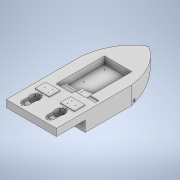
# Autodesk Inventor part: MainBody
Saved by Autodesk Inventor 2020.1 (Build 241239000, 239)
## iProperties
Created: 2021-12-15
Part Number: MainBody
Material: Generic
Document SubType Name: Modeling
Designer: OEM
Density: 1 g/cm^3
Appearance: Default
Author: OEM
Autodesk Inventor part; units mm, degrees
ref_plane "YZ Plane" through (0, 0, 0) normal (1, 0, 0) x (0, 1, 0)
ref_plane "XZ Plane" through (0, 0, 0) normal (0, 1, 0) x (-1, 0, 0)
ref_plane "XY Plane" through (0, 0, 0) normal (0, 0, 1) x (1, 0, 0)
sketch "Sketch1" plane through (0, 0, 0) normal (0, 1, 0) x (-1, 0, 0)
  line L0 (28.25, 20.4) -> (-28.25, 20.4) construction
  line L1 (-28.25, 20.4) -> (-28.25, -65.2) construction
  line L2 (-28.25, -65.2) -> (28.25, -65.2) construction
  line L3 (28.25, -65.2) -> (28.25, 20.4) construction
  line L4 (28.25, 20.4) -> (-28.25, -65.2) construction
  line L5 (-28.25, 20.4) -> (28.25, -65.2) construction
  line L6 (0, 600.8) -> (0, -638.2) construction
  spline S0 degree 2 poles (70, -42.8) (58.3679, -124.7541) (0, -160.2) knots 0 0 0 1 1 1
  line L7 (70, -42.8) -> (70, 157.2)
  spline S1 degree 2 poles (-70, -42.8) (-58.3679, -124.7541) (0, -160.2) knots 0 0 0 1 1 1
  line L8 (-70, -42.8) -> (-70, 157.2)
  line L9 (70, 87.2) -> (-70, 87.2)
  line L10 (0, 87.2) -> (70, 157.2) construction
  line L11 (0, 157.2) -> (70, 87.2) construction
  circle A0 centre (35, 122.2) radius 12.5
  line L12 (0, 87.2) -> (-70, 157.2) construction
  line L13 (0, 157.2) -> (-70, 87.2) construction
  circle A1 centre (-35, 122.2) radius 12.5
  line L14 (-38.25, 30.4) -> (38.25, 30.4)
  line L15 (38.25, 30.4) -> (38.25, -75.2)
  line L16 (38.25, -75.2) -> (-38.25, -75.2)
  line L17 (-38.25, -75.2) -> (-38.25, 30.4)
  line L18 (-38.25, 30.4) -> (38.25, -75.2) construction
  line L19 (38.25, 30.4) -> (-38.25, -75.2) construction
  line L20 (-6.75, 50.4) -> (38.25, 50.4)
  line L21 (38.25, 50.4) -> (38.25, 30.4)
  line L22 (-6.75, 30.4) -> (-6.75, 50.4)
  circle A2 centre (24.5, -61.7) radius 1.125
  circle A3 centre (-24.5, -61.7) radius 1.125
  line L23 (-24.5, -61.7) -> (24.5, -61.7) construction
  line L24 (-24.5, -32.7) -> (24.5, -32.7) construction
  line L25 (-24.5, -32.7) -> (-24.5, -61.7) construction
  line L26 (24.5, -32.7) -> (24.5, -61.7) construction
  circle A4 centre (24.5, -3.7) radius 1.125
  circle A5 centre (-24.5, -3.7) radius 1.125
  line L27 (-24.5, -3.7) -> (24.5, -3.7) construction
  line L28 (-24.5, -32.7) -> (-24.5, -3.7) construction
  line L29 (24.5, -32.7) -> (24.5, -3.7) construction
  line L30 (-6.75, 30.4) -> (-38.25, 30.4)
  line L31 (-38.25, 30.4) -> (-38.25, 50.4) construction
  line L32 (-38.25, 50.4) -> (-6.75, 50.4) construction
  line L33 (-6.75, 50.4) -> (-6.75, 30.4)
  line L34 (-6.75, 30.4) -> (-37.23, 30.4)
  line L35 (-37.23, 30.4) -> (-37.23, 51.99)
  line L36 (-37.23, 51.99) -> (-6.75, 51.99)
  line L37 (-6.75, 51.99) -> (-6.75, 30.4)
  circle A6 centre (-34.69, 32.94) radius 0.75
  circle A7 centre (-20.085, 49.45) radius 0.75
  line L38 (-45, 112.2) -> (-45, 152)
  line L39 (-45, 152) -> (-25, 152)
  line L40 (-25, 112.2) -> (-25, 108.45) construction
  line L41 (-25, 108.45) -> (-45, 108.45) construction
  line L42 (-45, 108.45) -> (-45, 112.2) construction
  line L43 (-25, 112.2) -> (-25, 152)
  line L44 (-45, 112.2) -> (-25, 112.2)
  line L45 (-25, 152) -> (-45, 152)
  line L46 (-45, 152) -> (-45, 155.75) construction
  line L47 (-45, 155.75) -> (-25, 155.75) construction
  line L48 (-25, 155.75) -> (-25, 152) construction
  line L49 (70, 157.2) -> (-70, 157.2) construction
  line L50 (-70, 157.2) -> (-70, 167.2)
  line L51 (-70, 167.2) -> (70, 167.2)
  line L52 (70, 167.2) -> (70, 157.2)
  line L53 (-35, 108.45) -> (-35, 155.75) construction
  circle A8 centre (-30, 155.75) radius 2
  line L54 (-25, 132.1) -> (-45, 132.1) construction
  circle A9 centre (-40, 155.75) radius 2
  circle A10 centre (-30, 108.45) radius 2
  circle A11 centre (-40, 108.45) radius 2
  line L55 (45, 112.2) -> (45, 152)
  line L56 (45, 152) -> (25, 152)
  line L57 (25, 112.2) -> (25, 152)
  line L58 (45, 112.2) -> (25, 112.2)
  line L59 (45, 152) -> (45, 155.75) construction
  line L60 (45, 155.75) -> (25, 155.75) construction
  line L61 (25, 155.75) -> (25, 152) construction
  line L62 (35, 108.45) -> (35, 155.75) construction
  circle A12 centre (30, 155.75) radius 2
  circle A13 centre (40, 155.75) radius 2
  circle A14 centre (30, 108.45) radius 2
  circle A15 centre (40, 108.45) radius 2
  line L63 (45, 108.45) -> (25, 108.45) construction
  line L64 (45, 108.45) -> (45, 112.2) construction
  line L65 (25, 108.45) -> (25, 112.2) construction
  line L66 (-72.4135, -25.7958) -> (-67.5865, -59.8042) construction
  arc A16 (-71.5687, -29.1646) -> (-67.7125, -56.3334) centre (186.925, -6.3334) ccw construction
  line L67 (-15, 102.2) -> (-55, 102.2)
  line L68 (-55, 102.2) -> (-55, 72.2)
  line L69 (-55, 72.2) -> (-15, 72.2)
  line L70 (-15, 72.2) -> (-15, 102.2)
  line L71 (-15, 102.2) -> (-55, 72.2) construction
  line L72 (-55, 102.2) -> (-15, 72.2) construction
  line L73 (15, 102.2) -> (55, 102.2)
  line L74 (55, 102.2) -> (55, 72.2)
  line L75 (55, 72.2) -> (15, 72.2)
  line L76 (15, 72.2) -> (15, 102.2)
  circle A17 centre (26.8629, 81.1136) radius 0.75
  circle A18 centre (42.4108, 87.2) radius 0.75
  circle A19 centre (26.8629, 93.2864) radius 0.75
  circle A20 centre (-26.8629, 81.1136) radius 0.75
  circle A21 centre (-42.4108, 87.2) radius 0.75
  circle A22 centre (-26.8629, 93.2864) radius 0.75
  line L77 (-26.75, 30.4) -> (-26.75, 33.4)
  line L78 (-26.75, 33.4) -> (-37.23, 33.4) construction
  line L79 (-14.75, 33.4) -> (-14.75, 51.99)
  line L80 (-14.75, 33.4) -> (-26.75, 33.4)
  line L81 (-14.75, 33.4) -> (-14.75, 30.4) construction
  line L82 (-14.75, 33.4) -> (-6.75, 33.4) construction
  line L83 (-37.23, 50.99) -> (-62.23, 50.99)
  line L84 (-37.23, 40.99) -> (-62.23, 40.99)
  line L85 (-62.23, 50.99) -> (-62.23, 40.99)
  line L86 (-35.6, 152) -> (-35.6, 160)
  line L87 (-35.6, 160) -> (-35, 160)
  line L88 (-34.4, 152) -> (-34.4, 160)
  line L89 (-34.4, 160) -> (-35, 160)
  line L90 (-35.6, 112.2) -> (-35.6, 104.2)
  line L91 (-35.6, 104.2) -> (-35, 104.2)
  line L92 (-34.4, 112.2) -> (-34.4, 104.2)
  line L93 (-34.4, 104.2) -> (-35, 104.2)
  line L94 (35.6, 152) -> (35.6, 160)
  line L95 (35.6, 160) -> (35, 160)
  line L96 (34.4, 152) -> (34.4, 160)
  line L97 (34.4, 160) -> (35, 160)
  line L98 (35.6, 112.2) -> (35.6, 104.2)
  line L99 (34.4, 112.2) -> (34.4, 104.2)
  line L100 (34.4, 104.2) -> (35, 104.2)
  line L101 (35.6, 104.2) -> (35, 104.2)
  point P0 (0, -22.4)
  point P1 (44.8, -116.1993)
  point P2 (-44.8, -116.1993)
  point P3 (25, 129.7)
  point P4 (45, 129.7)
  point P5 (27.5, 112.2)
  point P6 (25, 114.7)
  point P7 (42.5, 112.2)
  point P8 (45, 114.7)
  point P9 (-42.5, 112.2)
  point P10 (-45, 114.7)
  point P11 (-27.5, 112.2)
  point P12 (-25, 114.7)
  point P13 (-25, 129.7)
  point P14 (-45, 129.7)
  point P15 (-35, 87.2)
  dimension "d1" = 85.6
  dimension "d5" = 25
  dimension "d6" = 10
  dimension "d7" = 10
  dimension "d17" = 89.6
  dimension "d29" = 56.5
  dimension "d30" = 70
  dimension "d32" = 20
  dimension "d37" = 3.5
  dimension "d40" = 2.25
  dimension "d48" = 21.59
  dimension "d49" = 30.48
  dimension "d50" = 1.5
  dimension "d51" = 2.54
  dimension "d52" = 2.54
  dimension "d53" = 2.54
  dimension "d54" = 14.605
  dimension "d63" = 3.75
  dimension "d64" = 10
  dimension "d66" = 3.75
  dimension "d68" = 39.8
  dimension "d69" = 90
  dimension "d70" = 20
  dimension "d71" = 10
  dimension "d72" = 10
  dimension "d74" = 5
  dimension "d75" = 4
  dimension "d76" = 19.9
  dimension "d82" = 247.4
  dimension "d83" = 130
  dimension "d86" = 70
  dimension "d87" = 10
  dimension "d88" = 85
  dimension "d90" = 10
  dimension "d95" = 140
  dimension "d96" = 73.3993
  dimension "d97" = 38.25
  dimension "d98" = 10
  dimension "d99" = 35.921
  dimension "d100" = 33.427
  dimension "d101" = 90
  dimension "d102" = 90
  dimension "d105" = 1.5
  dimension "d106" = 6.0864
  dimension "d107" = 11.8628
  dimension "d108" = 1.5
  dimension "d109" = 15.548
  dimension "d115" = 1.5
  dimension "d117" = 58
  dimension "d120" = 24.5
  dimension "d121" = 24.5
  dimension "d122" = 37.23
  dimension "d126" = 20
  dimension "d136" = 1
  dimension "d137" = 25
  dimension "d138" = 10
  dimension "d141" = 0.6
  constraints: 204 end point, 48 symmetric about line, 23 centre point, 16 parallel, 16 point on line, 14 midpoint, 12 perpendicular, 11 horizontal, 7 vertical, 1 point on circle, 24 other
  measures "d1" distance of L1.end L0.end
  measures "d5" diameter of A0
  measures "d6" distance between parallel lines of L14 L0
  measures "d7" distance between parallel lines of L15 L3
  measures "d17" diameter of point (44.8, -116.199) L6
  measures "d29" distance between parallel lines of L1 L3
  measures "d30" distance between parallel lines of L6 L7
  measures "d32" distance between parallel lines of L14 L20
  measures "d37" distance from line of L2 A2.centre
  measures "d40" diameter of A2
  measures "d48" distance of L34.end L35.end
  measures "d49" distance of L35.end L36.end
  measures "d50" diameter of A6
  measures "d51" distance from line of L35 A6.centre
  measures "d52" distance from line of L14 A6.centre
  measures "d53" distance from line of L36 A7.centre
  measures "d54" horizontal distance of A6.centre A7.centre
  measures "d63" distance of L41.end L38.start
  measures "d64" horizontal distance of A1.centre L38.start
  measures "d66" distance of L38.end L46.end
  measures "d68" distance of L40.start L39.end
  measures "d69" angle of L38 L45
  measures "d70" distance of L40.end L41.end
  measures "d71" distance from line of L38 A1.centre
  measures "d72" distance from line of L43 A1.centre
  measures "d74" distance from line of L53 A8.centre
  measures "d75" diameter of A8
  measures "d76" distance of L40.start L54.start
  measures "d82" distance from line of L9 point (0, -160.2)
  measures "d83" distance of L9.end L8.start
  measures "d86" distance of L9.end L8.end
  measures "d87" distance of L49.end L50.end
  measures "d88" distance from line of point (0, -160.2) L16
  measures "d90" distance between parallel lines of L17 L1
  measures "d95" distance of L7.start L8.start
  measures "d96" vertical distance of L8.start point (-44.8, -116.199)
  measures "d97" distance between parallel lines of L15 L6
  measures "d98" distance between parallel lines of L16 L2
  measures "d99" angle of L15 L18
  measures "d100" angle of L3 L5
  measures "d101" angle of L23 L25
  measures "d102" angle of L23 L26
  measures "d105" diameter of A17
  measures "d106" distance from line of L9 A17.centre
  measures "d107" distance from line of L76 A17.centre
  measures "d108" diameter of A18
  measures "d109" horizontal distance of A17.centre A18.centre
  measures "d115" diameter of A7
  measures "d117" distance between parallel lines of L27 L23
  measures "d120" distance between parallel lines of L25 L6
  measures "d121" distance between parallel lines of L26 L6
  measures "d122" distance between parallel lines of L6 L35
  measures "d126" distance between parallel lines of L22 L77
  measures "d136" distance between parallel lines of L36 L83
  measures "d137" distance of L83.start L83.end
  measures "d138" distance between parallel lines of L83 L84
  measures "d141" distance between parallel lines of L53 L86
extrude "Body_front" add sketch "Sketch1" against normal blind 50 contours S0 S1 L8 L9 L68 L69 L70 L76 L75 L74 L7 | L74 L75 L76 L9 A18 | A18 L9 | L9 A21 L70 L69 L68 | L9 A21 | L14 L15 L16 L17 | L35 L36 L79 L80 L77 L14 | L77 L80 L79 L36 L37 L22 L14 | L84 L85 L83 L35 | L22 L20 L21 L14 | A2 | A3 | A4 | A5 | A6 | A7 | A17 | A20 picked at (42.4409, 86.9518) picked at (-42.3807, 86.9518)
extrude "Body_back" add sketch "Sketch1" against normal blind 20 contours S0 S1 L8 L9 L68 L69 L70 L76 L75 L74 L7 | L9 L74 L73 L76 L70 L67 L68 L8 L50 L51 L52 L7 | L74 L75 L76 L9 A18 | L9 A18 L76 L73 L74 | A18 L9 | L9 A18 | L68 L67 L70 L9 A21 | L9 A21 L70 L69 L68 | A21 L9 | L9 A21 | A0 L55 | L55 A0 L58 L57 | A0 L57 L56 L55 | L55 L58 A0 | L57 A0 | A0 L98 L58 | A0 L58 L57 | L56 L96 L97 L95 L94 | L98 L101 L100 L99 A0 | A0 L99 L58 L98 | L58 L99 A0 | A1 L43 | L43 A1 L44 L38 | A1 L38 L39 L43 | L43 L44 A1 | L38 A1 | A1 L92 L44 | A1 L44 L38 | L39 L86 L87 L89 L88 | L92 L93 L91 L90 A1 | A1 L90 L44 L92 | L44 L90 A1 | L14 L15 L16 L17 | L35 L36 L79 L80 L77 L14 | L77 L80 L79 L36 L37 L22 L14 | L84 L85 L83 L35 | L22 L20 L21 L14 | A2 | A3 | A4 | A5 | A6 | A7 | A8 | A9 | A10 | A11 | A12 | A13 | A14 | A15 | A17 | A19 | A20 | A22
extrude "RPi" cut sketch "Sketch1" against normal blind 20 contours L14 L15 L16 L17 | A2 | A3 | A4 | A5
extrude "RPI_USB" cut sketch "Sketch1" against normal blind 10 contours L22 L20 L21 L14
fillet "Fillet1" radius 10 1 edges at (-15.75, -10, 30.4)
fillet "Fillet2" radius 10 1 edges at (-15.75, 0, 50.4) inverted yes
extrude "RPi_mounting_holes" cut sketch "Sketch1" against normal blind 26 contours A2 | A3 | A4 | A5
extrude "Maestro" cut sketch "Sketch1" against normal blind 2 contours L35 L36 L79 L80 L77 L14 | L77 L80 L79 L36 L37 L22 L14
extrude "Maestro_mounting_holes" cut sketch "Sketch1" against normal blind 6 contours A6 | A7
extrude "Servo_body" cut sketch "Sketch1" against normal blind 7 contours A0 L57 L56 L55 | L55 L58 A0 | A0 L58 L57 | A1 L38 L39 L43 | L43 L44 A1 | A1 L44 L38
extrude "Servo_mounting_holes" cut sketch "Sketch1" against normal blind 10 contours A8 | A9 | A10 | A11 | A12 | A13 | A14 | A15
extrude "Engine_controller_holders" add sketch "Sketch1" along normal blind 2 contours L74 L75 L76 L9 A18 | L9 A18 L76 L73 L74 | A18 L9 | L9 A18 | L68 L67 L70 L9 A21 | L9 A21 L70 L69 L68 | A21 L9 | L9 A21 | A17 | A19 | A20 | A22
extrude "Motor_Controller_mounting_holes" cut sketch "Sketch1" along normal blind 2 and the other way blind 4 contours A18 L9 | L9 A18 | A21 L9 | L9 A21 | A17 | A19 | A20 | A22
extrude "maestro_pins_back" cut sketch "Sketch1" against normal blind 3 contours L77 L80 L79 L36 L37 L22 L14
extrude "Servo_sleeve" cut sketch "Sketch1" against normal blind 20 contours A0 L55 | L55 A0 L58 L57 | L57 A0 | A0 L98 L58 | A0 L99 L58 L98 | L58 L99 A0 | A1 L43 | L43 A1 L44 L38 | L38 A1 | A1 L92 L44 | A1 L90 L44 L92 | L44 L90 A1
sketch "Sketch7" plane through (70, -50, -42.8) normal (1, 0, 0) x (0, 0, -1)
  line L0 (0, 0) -> (-130, 0) projected
  line L1 (0, 0) -> (89, 11) construction
  line L2 (89, 11) -> (117.4, 50) construction
  spline S0 degree 2 poles (0, 0) (89, 11) (117.4, 50) knots 1 1 1 2 2 2
  line L3 (117.4, 50) -> (117.4, 0) projected
  line L4 (117.4, 50) -> (117.4, 0)
  line L5 (0, 50) -> (0, 0) projected
  line L6 (117.4, 0) -> (0, 0)
  circle A0 centre (8, 8) radius 3.5
  point P0 (-42.8, 50)
  dimension "d132" = 7
  constraints: 4 end point, 1 centre point, 1 perpendicular, 1 vertical, 3 other
  measures "d132" diameter of A0
extrude "Side_extrusion" cut sketch "Sketch7" against normal blind 150
extrude "maestro_USB" cut sketch "Sketch1" against normal blind 3 contours L84 L85 L83 L35
extrude "servo_traingle" cut sketch "Sketch1" against normal blind 3 contours L56 L96 L97 L95 L94 | L98 L101 L100 L99 A0 | A0 L99 L58 L98 | L39 L86 L87 L89 L88 | L92 L93 L91 L90 A1 | A1 L90 L44 L92
sketch "Sketch8" plane through (-70, -50, 87.2) normal (0, 0, 1) x (1, 0, 0)
  point P0 (70, 50)
  point P1 (67.4391, 21.974)
hole "Hole1" at (-2.5609, -28.026, 87.2) direction (0, 0, -1) diameter 10 depth 170.4942 tip angle 118
equation "\"d71\" = 0.5 * d70"
equation "\"d72\" = 0.5 * d70"
equation "\"d76\" = 0.5 * d68"
body "Solid1"
